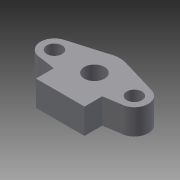
# Autodesk Inventor part: shaft support
Saved by Autodesk Inventor 2015 SP1 (Build 190203100, 203)
## iProperties
Created: 2016-07-11
Part Number: shaft support
Material: Generic
Document SubType Name: Modeling
Designer: lustinga
Density: 1 g/cm^3
Appearance: Default
Mass: 5.73387 g
Surface Area: 29.0478 cm^2
Volume: 5.73387 cm^3
Author: lustinga
Autodesk Inventor part; units mm, degrees
ref_plane "YZ Plane" through (0, 0, 0) normal (1, 0, 0) x (0, 1, 0)
ref_plane "XZ Plane" through (0, 0, 0) normal (0, 1, 0) x (-1, 0, 0)
ref_plane "XY Plane" through (0, 0, 0) normal (0, 0, 1) x (1, 0, 0)
sketch "Sketch1" plane through (0, 0, 0) normal (0, 0, 1) x (1, 0, 0)
  circle A0 centre (50.3282, 23.2015) radius 3
  circle A1 centre (18.8282, 23.2015) radius 3
  circle A2 centre (34.5782, 23.2015) radius 4
  arc A3 (37.4648, 32.7758) -> (30.5806, 32.3677) centre (34.5782, 23.2015) ccw
  arc A4 (50.3282, 17.7015) -> (51.8996, 28.4722) centre (50.3282, 23.2015) ccw
  line L0 (37.4648, 32.7758) -> (51.8996, 28.4722)
  line L1 (34.3282, 9.7015) -> (44.1532, 9.7015)
  line L2 (44.1532, 9.7015) -> (44.1532, 16.7015)
  line L3 (44.1532, 16.7015) -> (50.3282, 17.7015)
  line L4 (30.5806, 32.3677) -> (17.2831, 28.48)
  line L5 (34.3282, 9.7015) -> (25.0032, 9.7015)
  line L6 (25.0032, 9.7015) -> (25.0032, 16.7015)
  line L7 (25.0032, 16.7015) -> (18.8282, 17.7015)
  arc A5 (17.2831, 28.48) -> (18.8282, 17.7015) centre (18.8282, 23.2015) ccw
  circle A6 centre (34.5782, 23.2015) radius 8.7313
  point P0 (0, 0)
  dimension "d0" = 31.5
  dimension "d1" = 6
  dimension "d2" = 8
  dimension "d3" = 15.75
  dimension "d4" = 20
  dimension "d5" = 11
  dimension "d7" = 9.825
  dimension "d8" = 7
  dimension "d9" = 11
  dimension "d12" = 17.4625
  dimension "d14" = 0
  constraints: 16 end point, 7 centre point, 6 point on circle, 4 coincident, 1 equal radius, 1 horizontal alignment, 1 perpendicular, 1 tangent
  measures "d0" distance of A1.centre A0.centre
  measures "d1" diameter of A0
  measures "d2" diameter of A2
  measures "d3" distance of A1.centre A2.centre
  measures "d4" diameter of A3
  measures "d5" diameter of A4
  measures "d7" distance of L1.start L1.end
  measures "d8" distance of L1.end L2.end
  measures "d9" diameter of A5
  measures "d12" diameter of A6
  measures "d14" vertical distance of A0.centre A3.centre
extrude "Extrusion1" add sketch "Sketch1" along normal blind 10 contours L0 A4 L3 L2 L1 L5 L6 L7 A5 L4 A3 | A6
body "Solid1"
